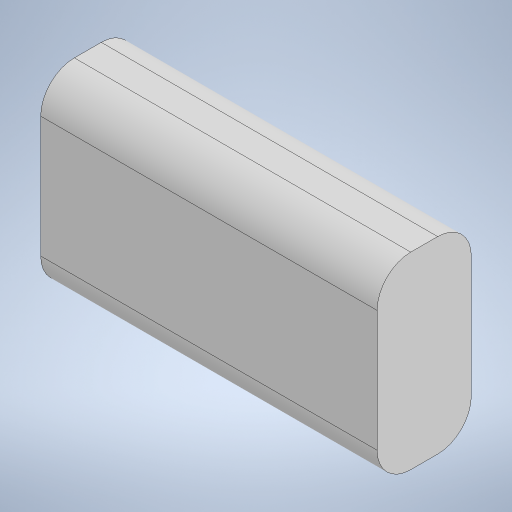
# Autodesk Inventor part: 7.4 V  500MaH Li pol
Saved by Autodesk Inventor 2023 (Build 270158000, 158)
## iProperties
Created: 2023-01-20
Part Number: 7.4 V  500MaH Li pol
Material: Všeobecné
Document SubType Name: Modeling
Designer: Kuba
Mass: 18.527 g
Surface Area: 45.1188 cm^2
Volume: 18.527 cm^3
Density: 1 g/cm^3
Appearance: Výchozí
Author: Kuba
Autodesk Inventor part; units mm, degrees
ref_plane "YZ Plane" through (0, 0, 0) normal (1, 0, 0) x (0, 1, 0)
ref_plane "XZ Plane" through (0, 0, 0) normal (0, 1, 0) x (-1, 0, 0)
ref_plane "XY Plane" through (0, 0, 0) normal (0, 0, 1) x (1, 0, 0)
sketch "Náčrt1" plane through (0, 0, 0) normal (0, 0, 1) x (1, 0, 0)
  line L0 (0, 0) -> (-25, 0) construction
  line L1 (-25, 0) -> (-25, -14) construction
  line L2 (-25, -14) -> (0, -14) construction
  line L3 (0, -14) -> (0, 0) construction
  line L4 (-25, -14) -> (25, -14)
  line L5 (25, -14) -> (25, 14)
  line L6 (25, 14) -> (-25, 14)
  line L7 (-25, 14) -> (-25, -14)
  dimension "d0" = 25
  dimension "d1" = 14
  dimension "d2" = 50
  dimension "d3" = 28
  constraints: 16 end point, 4 parallel, 2 horizontal, 2 perpendicular
  measures "d0" distance of L2.end L1.end
  measures "d1" distance of L1.end L0.end
  measures "d2" distance of L6.end L5.end
  measures "d3" distance of L5.end L4.end
extrude "Vysunutí1" add sketch "Náčrt1" along normal blind 14
fillet "Zaoblení1" radius 5 4 edges at (0, 14, 14) (0, 14, 0) (0, -14, 14) (0, -14, 0)
